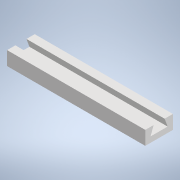
# Autodesk Inventor part: prismatic link inner
Saved by Autodesk Inventor 2021 (Build 250183000, 183)
## iProperties
Created: 2022-03-22
Part Number: prismatic link inner
Material: Generic
Document SubType Name: Modeling
Designer: techv
Density: 1 g/cm^3
Appearance: Default
Author: techv
Autodesk Inventor part; units mm, degrees
ref_plane "YZ Plane" through (0, 0, 0) normal (1, 0, 0) x (0, 1, 0)
ref_plane "XZ Plane" through (0, 0, 0) normal (0, 1, 0) x (-1, 0, 0)
ref_plane "XY Plane" through (0, 0, 0) normal (0, 0, 1) x (1, 0, 0)
sketch "Sketch1" plane through (0, 0, 0) normal (1, 0, 0) x (0, 1, 0)
  line L0 (-5, 10) -> (5, 10)
  line L1 (5, 10) -> (5, -10)
  line L2 (5, -10) -> (-5, -10)
  line L3 (-5, -10) -> (-5, 10)
  line L4 (-5, 10) -> (5, -10) construction
  line L5 (5, 10) -> (-5, -10) construction
  line L6 (-1, 6.1838) -> (-1, -6.1838)
  line L7 (-1, -6.1838) -> (5, -4)
  line L8 (-1, 6.1838) -> (5, 4)
  point P0 (0, 0)
  dimension "d0" = 10
  dimension "d1" = 20
  dimension "d3" = 110
  dimension "d4" = 110
  dimension "d5" = 6
  dimension "d6" = 6
  dimension "d7" = 6
  dimension "d8" = 6
  constraints: 18 end point, 2 midpoint, 2 parallel, 2 point on line, 1 horizontal, 1 perpendicular
  measures "d0" distance of L1.end L2.end
  measures "d1" distance of L0.end L1.end
  measures "d3" angle of L8 L1
  measures "d4" angle of L1 L7
  measures "d5" horizontal distance of L6.end L7.end
  measures "d6" horizontal distance of L6.start L8.end
  measures "d7" distance of L0.end L8.end
  measures "d8" distance of L1.end L7.end
extrude "Extrusion1" add sketch "Sketch1" along normal blind 100 contours L0 L1 L8 L6 L7 L2 L3
sketch "Sketch2" plane through (0, 0, 0) normal (-1, 0, 0) x (0, 0, 1)
  line L0 (-10, -5) -> (-10, 5) projected
  line L1 (-10, -5) -> (10, -5)
  line L2 (10, -5) -> (10, 9)
  line L3 (10, 9) -> (-10, 9)
  line L4 (-10, 9) -> (-10, -5)
  point P0 (0, 0)
  dimension "d11" = 20
  dimension "d12" = 14
  constraints: 8 end point, 2 parallel, 1 horizontal, 1 perpendicular
  measures "d11" distance of L3.end L2.end
  measures "d12" distance of L2.end L1.end
extrude "Extrusion2" add sketch "Sketch2" along normal blind 3
sketch "Sketch3" plane through (100, -5, -10) normal (0, -1, 0) x (1, 0, 0)
  circle A0 centre (-6, 10) radius 1.5 projected
  circle A1 centre (-14, 10) radius 1.5 projected
  circle A2 centre (-22, 10) radius 1.5 projected
  circle A3 centre (-30, 10) radius 1.5 projected
  circle A4 centre (-38, 10) radius 1.5 projected
  circle A5 centre (-46, 10) radius 1.5 projected
  circle A6 centre (-54, 10) radius 1.5 projected
  line L0 (-103, 0) -> (0, 0) projected
  line L1 (0, 20) -> (0, 0) projected
  line L2 (0, 20) -> (-103, 20) projected
  line L3 (-103, 0) -> (-103, 20) projected
  circle A7 centre (-62, 10) radius 1.5 projected
  circle A8 centre (-70, 10) radius 1.5 projected
  circle A9 centre (-78, 10) radius 1.5 projected
  circle A10 centre (-86, 10) radius 1.5 projected
  circle A11 centre (-94, 10) radius 1.5 projected
  point P0 (-100, 10)
extrude "Extrusion3" cut sketch "Sketch3" against normal through all contours A0 | A1 | A2 | A3 | A4 | A5 | A6 | A7 | A8 | A9 | A10 | A11
body "Solid1"
